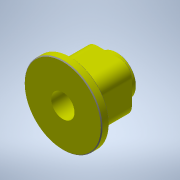
# Autodesk Inventor part: Front_bush
Saved by Autodesk Inventor 2020 (Build 240168000, 168)
## iProperties
Created: 2015-12-03
Part Number: Front_bush
Material: Genérico
Document SubType Name: Modeling
Designer: MIGUEL ANGEL
Density: 1 g/cm^3
Appearance: Valor por defecto
Author: MIGUEL ANGEL
Autodesk Inventor part; units mm, degrees
ref_plane "YZ Plane" through (0, 0, 0) normal (1, 0, 0) x (0, 1, 0)
ref_plane "XZ Plane" through (0, 0, 0) normal (0, 1, 0) x (-1, 0, 0)
ref_plane "XY Plane" through (0, 0, 0) normal (0, 0, 1) x (1, 0, 0)
sketch "Boceto1" plane through (0, 0, 0) normal (0, 1, 0) x (-1, 0, 0)
  circle A0 centre (0, 0) radius 10
  dimension "d0" = 20
  constraints: 1 centre point, 1 coincident
  measures "d0" diameter of A0
extrude "Extrusión1" add sketch "Boceto1" along normal blind 2
sketch "Boceto2" plane through (0, 2, 0) normal (0, 1, 0) x (1, 0, 0)
  line L0 (-3, -6) -> (3, -6)
  line L1 (6, -3) -> (6, 3)
  line L2 (3, 6) -> (-3, 6)
  line L3 (-6, 3) -> (-6, -3)
  arc A0 (-3, 6) -> (-6, 3) centre (-3, 3) ccw
  arc A1 (-6, -3) -> (-3, -6) centre (-3, -3) ccw
  arc A2 (3, -6) -> (6, -3) centre (3, -3) ccw
  arc A3 (6, 3) -> (3, 6) centre (3, 3) ccw
  point P0 (0, 0)
  point P1 (-6, -6)
  point P2 (6, 6)
  point P3 (-6, 6)
  point P4 (0, 6)
  point P5 (-6, 0)
  dimension "d3" = 12
  dimension "d4" = 12
  dimension "d5" = 3
  constraints: 8 end point, 8 point on circle, 8 tangent, 6 point on line, 4 centre point, 3 equal radius, 2 midpoint, 2 parallel, 1 horizontal, 1 horizontal alignment, 1 perpendicular, 1 vertical alignment
  measures "d3" distance of point (-6, 6) point (-6, -6)
  measures "d4" distance of point (6, 6) point (-6, 6)
  measures "d5" radius of A0
extrude "Extrusión2" add sketch "Boceto2" along normal blind 10
sketch "Boceto3" plane through (0, 12, 0) normal (0, 1, 0) x (1, 0, 0)
  circle A0 centre (0, 0) radius 5
  dimension "d8" = 10
  constraints: 1 centre point, 1 coincident
  measures "d8" diameter of A0
extrude "Extrusión3" add sketch "Boceto3" along normal blind 2
sketch "Boceto4" plane through (0, 0, 0) normal (0, -1, 0) x (1, 0, 0)
  circle A0 centre (0, 0) radius 3
  dimension "d11" = 6
  constraints: 1 centre point, 1 coincident
  measures "d11" diameter of A0
extrude "Extrusión4" cut sketch "Boceto4" against normal blind 12
chamfer "Chaflán1" distance 0.2 angle 45 11 edges at (-5, 14, 0) (6, 12, 0) (5.1213, 12, -5.1213) (0, 12, -6) (-5.1213, 12, -5.1213) (-6, 12, 0) (-5.1213, 12, 5.1213) (0, 12, 6) (5.1213, 12, 5.1213) (10, 2, 0) (10, 0, 0)
